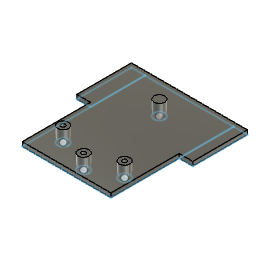
MCU-standoff (Autodesk Fusion 360 design; units mm, degrees)
Autodesk Fusion 360 part; units mm, degrees
sketch "Sketch1" plane through (0, 0, 0) normal (0, 0, 1) x (1, 0, 0)
  line L0 (-52.7867, 65.4525) -> (-19.7667, 65.4525)
  line L1 (-19.7667, 65.4525) -> (-19.7667, 19.7325)
  line L2 (-19.7667, 19.7325) -> (-52.7867, 19.7325)
  line L3 (-52.7867, 19.7325) -> (-52.7867, 65.4525)
  line L4 (-19.7667, 65.4525) -> (-14.6867, 65.4525)
  line L5 (-14.6867, 65.4525) -> (-14.6867, 45.1325)
  line L6 (-14.6867, 45.1325) -> (-19.7667, 45.1325)
  line L7 (-19.7667, 45.1325) -> (-19.7667, 65.4525)
  line L8 (-52.7867, 65.4525) -> (-57.8667, 65.4525)
  line L9 (-57.8667, 65.4525) -> (-57.8667, 45.1325)
  line L10 (-57.8667, 45.1325) -> (-52.7867, 45.1325)
  line L11 (-52.7867, 45.1325) -> (-52.7867, 65.4525)
  circle A0 centre (-23.5767, 28.6225) radius 0.8
  circle A1 centre (-23.5767, 28.6225) radius 2
  circle A2 centre (-46.4367, 28.6225) radius 0.8
  circle A3 centre (-46.4367, 28.6225) radius 2
  circle A4 centre (-33.7367, 23.5425) radius 0.8
  circle A5 centre (-33.7367, 23.5425) radius 2
  circle A6 centre (-37, 55) radius 2
  dimension "d3" = 33.02
  dimension "d4" = 45.72
  dimension "d5" = 5.08
  dimension "d6" = 20.32
  dimension "d7" = 5.08
  dimension "d8" = 20.32
  dimension "d9" = 1.6
  dimension "d10" = 4
  dimension "d11" = 3.81
  dimension "d12" = 1.6
  dimension "d13" = 4
  dimension "d14" = 22.86
  dimension "d15" = 1.6
  dimension "d16" = 4
  dimension "d17" = 5.08
  dimension "d18" = 10.16
  dimension "d19" = 8.89
  dimension "d20" = 8.89
  dimension "d25" = 4
  constraint horizontal L0
  constraint vertical L1
  constraint horizontal L2
  constraint vertical L3
  constraint horizontal L4
  constraint vertical L5
  constraint horizontal L6
  constraint vertical L7
  constraint horizontal L8
  constraint vertical L9
  constraint horizontal L10
  constraint vertical L11
  constraint concentric A0 A1
  constraint concentric A2 A3
  constraint concentric A4 A5
  measures "d3" distance of L0.start L0.end
  measures "d4" distance of L0.start L2.end
  measures "d5" distance of L0.end L4.end
  measures "d6" distance of L0.end L6.end
  measures "d7" distance of L0.start L8.end
  measures "d8" distance of L0.start L10.end
  measures "d9" diameter of A0
  measures "d10" diameter of A1
  measures "d11" distance of L1 A0.centre
  measures "d12" diameter of A2
  measures "d13" diameter of A3
  measures "d14" horizontal distance of A0.centre A2.centre
  measures "d15" diameter of A4
  measures "d16" diameter of A5
  measures "d17" vertical distance of A0.centre A4.centre
  measures "d18" horizontal distance of A0.centre A4.centre
  measures "d19" distance of L2 A0.centre
  measures "d20" distance of L2 A2.centre
  measures "d25" diameter of A6
extrude "Extrude1" add sketch "Sketch1" along normal blind 1.5 contours L0 L1 L2 L3 L7 L11 | L3 L8 L9 L10 L11 | L1 L4 L5 L6 L7 | A0 | A1 | A2 | A3 | A4 | A5 | A6 makes body 1
extrude "Extrude2" add sketch "Sketch1" along normal blind 5.5 separate body contours A1 | A3 | A5 makes body 2 at (-44.4392, 28.5228, 3.6667) makes body 3 at (-31.7392, 23.4428, 3.6667) makes body 4 at (-21.5792, 28.5228, 3.6667)
extrude "Extrude3" add sketch "Sketch1" along normal blind 5.5 separate body contours A6 makes body 5
